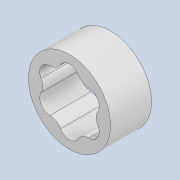
# Autodesk Inventor part: 2ギア接続部外
Saved by Autodesk Inventor 2020.4 (Build 244396000, 396)
## iProperties
Created: 2021-04-23
Part Number: 2ギア接続部外
Material: アルミニウム 2014-T4
Document SubType Name: Modeling
Designer: happy
Density: 2.8 g/cm^3
Appearance: サテン
Author: happy
Autodesk Inventor part; units mm, degrees
ref_plane "YZ Plane" through (0, 0, 0) normal (1, 0, 0) x (0, 1, 0)
ref_plane "XZ Plane" through (0, 0, 0) normal (0, 1, 0) x (-1, 0, 0)
ref_plane "XY Plane" through (0, 0, 0) normal (0, 0, 1) x (1, 0, 0)
sketch "スケッチ1" plane through (0, 0, 0) normal (0, 0, 1) x (1, 0, 0)
  arc A0 (69.7697, -24.216) -> (68.6872, -22.341) centre (68.6872, -23.591) ccw
  arc A1 (69.7697, -24.216) -> (69.7697, -25.716) centre (71.0687, -24.966) ccw
  arc A2 (68.6872, -27.591) -> (69.7697, -25.716) centre (68.6872, -26.341) ccw
  arc A3 (65.2231, -28.341) -> (67.3881, -28.341) centre (66.3056, -27.716) ccw
  arc A4 (68.6872, -27.591) -> (67.3881, -28.341) centre (68.6872, -29.091) ccw
  arc A5 (65.2231, -28.341) -> (63.924, -27.591) centre (63.924, -29.091) ccw
  arc A6 (63.924, -22.341) -> (62.8415, -24.216) centre (63.924, -23.591) ccw
  arc A7 (63.924, -22.341) -> (65.2231, -21.591) centre (63.924, -20.841) ccw
  line L0 (62.8415, -22.966) -> (66.3056, -20.966) construction
  circle A8 centre (66.3056, -24.966) radius 5
  arc A9 (67.3881, -21.591) -> (65.2231, -21.591) centre (66.3056, -22.216) ccw
  arc A10 (62.8415, -25.716) -> (62.8415, -24.216) centre (61.5425, -24.966) ccw
  arc A11 (67.3881, -21.591) -> (68.6872, -22.341) centre (68.6872, -20.841) ccw
  line L1 (62.8415, -26.966) -> (62.8415, -22.966) construction
  arc A12 (62.8415, -25.716) -> (63.924, -27.591) centre (63.924, -26.341) ccw
  line L2 (66.3056, -20.966) -> (69.7697, -22.966) construction
  line L3 (66.3056, -28.966) -> (62.8415, -26.966) construction
  circle A13 centre (66.3056, -24.966) radius 4 construction
  circle A14 centre (66.3056, -24.966) radius 3.2631 construction
  line L4 (69.7697, -26.966) -> (66.3056, -28.966) construction
  line L5 (69.7697, -22.966) -> (69.7697, -26.966) construction
  point P0 (0, 0)
  point P1 (69.7697, -26.966)
  point P2 (66.3056, -28.966)
  point P3 (65.2231, -28.341)
  point P4 (63.924, -27.591)
  point P5 (62.8415, -25.716)
  point P6 (63.924, -22.341)
  point P7 (69.7697, -24.216)
  point P8 (69.7697, -25.716)
  point P9 (68.6872, -27.591)
  dimension "d5" = 8
  dimension "d4" = 10
  dimension "d6" = 360
  dimension "d7" = 360
  dimension "d8" = 6.5263
  dimension "d9" = 1.5
  dimension "d10" = 1.25
  constraints: 30 point on circle, 14 centre point, 12 end point, 3 coincident, 2 point on line, 2 tangent, 1 vertical, 1 vertical alignment, 73 other
  measures "d4" diameter of A8
  measures "d8" diameter of A14
  measures "d9" radius of A11
  measures "d10" radius of A9
extrude "押し出し1" add sketch "スケッチ1" along normal blind 5
